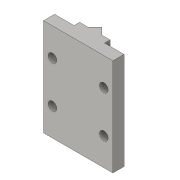
# Autodesk Inventor part: Oberstempel_2016_iLogic
Saved by Autodesk Inventor 2016 (Build 200138000, 138)
## iProperties
Created: 2015-09-14
Part Number: Oberstempel_2016_iLogic
Material: Generisch
Document SubType Name: Modeling
Designer: bauermeisterdi
Density: 1 g/cm^3
Appearance: Vorgabe
Author: bauermeisterdi
Autodesk Inventor part; units mm, degrees
ref_plane "YZ Plane" through (0, 0, 0) normal (1, 0, 0) x (0, 1, 0)
ref_plane "XZ Plane" through (0, 0, 0) normal (0, 1, 0) x (-1, 0, 0)
ref_plane "XY Plane" through (0, 0, 0) normal (0, 0, 1) x (1, 0, 0)
sketch "Skizze_Grundkörper" plane through (0, 0, 0) normal (0, 0, 1) x (1, 0, 0)
  line L0 (-35, 0) -> (35, 0) projected
  line L1 (0, -3.4) -> (0, 20.4) projected
  line L2 (-25, 0) -> (25, 0)
  line L3 (25, 0) -> (25, 8)
  line L4 (25, 8) -> (11, 8)
  line L5 (11, 8) -> (11, 12)
  line L6 (11, 12) -> (5, 12)
  line L7 (5, 12) -> (0, 17)
  line L8 (0, 17) -> (-5, 12)
  line L9 (-5, 12) -> (-11, 12)
  line L10 (-11, 12) -> (-11, 8)
  line L11 (-11, 8) -> (-25, 8)
  line L12 (-25, 8) -> (-25, 0)
  point P0 (0, 0)
  dimension "Breite" = 50
  dimension "Absatzbreite" = 22
  dimension "Absatzhöhe" = 8
  dimension "Absatz" = 12
  dimension "Höhe" = 17
  dimension "Winkel" = 90
  constraints: 22 end point, 4 vertical, 3 collinear, 3 horizontal, 1 parallel, 1 point on line, 3 other
  measures "Breite" distance between parallel lines of L3 L12
  measures "Absatzbreite" distance between parallel lines of L5 L10
  measures "Absatzhöhe" distance of L11.end L2.start
  measures "Absatz" distance between parallel lines of L6 L2
  measures "Höhe" distance from line of L7.end L2
  measures "Winkel" angle of L7 L8
extrude "Grundkörper" add sketch "Skizze_Grundkörper" along normal mid plane 70
sketch "Skizze_Bohrung" plane through (11, 8, 35) normal (0, 1, 0) x (1, 0, 0)
  line L0 (-46, 35) -> (24, 35) projected
  line L1 (-11, 84) -> (-11, -14) projected
  point P0 (-11, 35)
  point P1 (-29.5, 50)
  point P2 (7.5, 50)
  point P3 (7.5, 20)
  point P4 (-29.5, 20)
  dimension "Abstandbreite_Bohrung" = 37
  dimension "Abstandlänge" = 30
  constraints: 3 symmetric about line
  measures "Abstandbreite_Bohrung" distance of point (7.5, 50) point (-29.5, 50)
  measures "Abstandlänge" distance of point (-29.5, 20) point (-29.5, 50)
hole "Bohrung" at (-18.5, 8, -15) at (18.5, 8, -15) at (18.5, 8, 15) at (-18.5, 8, 15) direction (0, -1, 0) diameter 6.2 end through all
